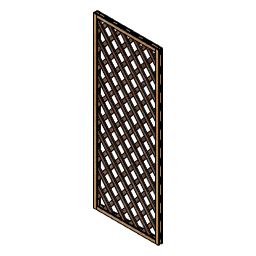
Latice Hanger (Autodesk Fusion 360 archive; units mm, degrees)
design "Lattice Wall"
Autodesk Fusion 360 part; units mm, degrees
sketch "Sketch1" plane through (0, 0, 0) normal (0, 1, 0) x (1, 0, 0) in component "Front"
  line L0 (405, 1050) -> (-405, 1050)
  line L1 (-405, 1050) -> (-405, -1050)
  line L2 (-405, -1050) -> (405, -1050)
  line L3 (405, -1050) -> (405, 1050)
  line L4 (405, 1050) -> (-405, -1050) construction
  line L5 (-405, 1050) -> (405, -1050) construction
  line L6 (-366, -1050) -> (-366, 1050)
  line L7 (0, -1645) -> (0, 1420) construction
  line L8 (366, -1050) -> (366, 1050)
  line L9 (366, -1011) -> (-366, -1011)
  line L10 (-366, 1011) -> (366, 1011)
  dimension "d2" = 810
  dimension "d3" = 2100
  dimension "d4" = 39
  dimension "d9" = 39
  dimension "d10" = 39
  constraint horizontal L0
  constraint perpendicular L0 L1
  constraint parallel L0 L2
  constraint parallel L1 L3
  constraint coincident L4 origin
  constraint coincident L5 origin
  constraint coincident L2 L6.start
  constraint coincident L0 L6.end
  constraint perpendicular L0 L6
  constraint perpendicular L2 L7
  constraint symmetric L6.start L7 L8.start
  constraint symmetric L6.end L7 L8.end
  constraint coincident L8 L9.start
  constraint coincident L6 L9.end
  constraint perpendicular L6 L9
  constraint coincident L6 L10.start
  constraint coincident L8 L10.end
  constraint perpendicular L8 L10
  measures "d2" distance of L1.end L2.end
  measures "d3" distance of L0.end L1.end
  measures "d4" distance of L1 L6
  measures "d9" distance of L2 L9
  measures "d10" distance of L0 L10
extrude "Extrude1" add sketch "Sketch1" along normal blind 12 contours L0 L2 L3 L8 | L0 L1 L2 L6 makes body 1 at (-392, 0, -350) makes body 2 at (379, 0, 350) in component "Front"
extrude "Extrude2" add sketch "Sketch1" along normal blind 12 separate body contours L0 L6 L8 L10 | L2 L6 L8 L9 makes body 3 at (-122, 0, -1024) makes body 4 at (-122, 0, 1037) in component "Front"
sketch "Sketch1 (2)" plane through (0, 0, 0) normal (0, 1, 0) x (1, 0, 0) in component "Middle Front"
  line L0 (-366, -1050) -> (-366, 1050) construction
  line L1 (366, -1011) -> (-366, -1011) construction
  line L2 (366, -1050) -> (366, 1050) construction
  line L3 (-366, 1011) -> (366, 1011) construction
  line L4 (-397.4531, -1050) -> (405, -55.0052)
  line L5 (405, 7.1195) -> (-405, -997.2331)
  line L6 (405, -190.405) -> (-288.2545, -1050)
  line L7 (-238.1517, -1050) -> (405, -252.5296)
  line L8 (80.4512, -1050) -> (405, -647.5785)
  line L9 (405, -585.4539) -> (30.3483, -1050)
  line L10 (-78.8502, -1050) -> (405, -450.054)
  line L11 (405, -387.9294) -> (-128.9531, -1050)
  line L12 (405, -1050) -> (405, 1050)
  line L13 (-405, -1050) -> (405, -1050)
  line L14 (-405, 1050) -> (-405, -1050)
  line L15 (405, 1050) -> (-405, 1050)
  line L16 (239.7526, -1050) -> (405, -845.1029)
  line L17 (405, -782.9783) -> (189.6497, -1050)
  line L18 (405, 204.6439) -> (-405, -799.7087)
  line L19 (-405, -861.8333) -> (405, 142.5193)
  line L20 (405, 402.1683) -> (-405, -602.1842)
  line L21 (-405, -664.3088) -> (405, 340.0437)
  line L22 (405, 599.6928) -> (-405, -404.6598)
  line L23 (-405, -466.7844) -> (405, 537.5682)
  line L24 (405, 797.2172) -> (-405, -207.1353)
  line L25 (-405, -269.26) -> (405, 735.0926)
  line L26 (405, 994.7417) -> (-405, -9.6109)
  line L27 (-405, -71.7355) -> (405, 932.617)
  line L28 (290.2639, 1050) -> (-405, 187.9135)
  line L29 (-405, 125.7889) -> (340.3667, 1050)
  line L30 (130.9624, 1050) -> (-405, 385.438)
  line L31 (-405, 323.3134) -> (181.0653, 1050)
  line L32 (-28.339, 1050) -> (-405, 582.9624)
  line L33 (-405, 520.8378) -> (21.7639, 1050)
  line L34 (-187.6404, 1050) -> (-405, 780.4869)
  line L35 (-405, 718.3622) -> (-137.5376, 1050)
  dimension "d15" = 39
  dimension "d16" = 39
  dimension "d17" = 85
  dimension "d18" = 39
  dimension "d19" = 39
  dimension "d20" = 85
  dimension "d21" = 85
  dimension "d22" = 39
  dimension "d23" = 85
  dimension "d24" = 39
  dimension "d25" = 39
  dimension "d26" = 39
  dimension "d27" = 39
  dimension "d28" = 39
  dimension "d29" = 39
  dimension "d30" = 39
  dimension "d31" = 39
  dimension "d32" = 39
  dimension "d33" = 85
  dimension "d34" = 85
  dimension "d35" = 85
  dimension "d36" = 85
  dimension "d37" = 85
  dimension "d38" = 85
  dimension "d39" = 85
  dimension "d40" = 85
  dimension "d41" = 85
  constraint parallel L4 L5
  constraint parallel L6 L7
  constraint parallel L10 L11
  constraint parallel L8 L9
  constraint coincident L12 L8.end
  constraint coincident L12 L9.start
  constraint coincident L12 L10.end
  constraint coincident L12 L11.start
  constraint coincident L12 L7.end
  constraint coincident L12 L6.start
  constraint coincident L12 L4.end
  constraint coincident L12 L5.start
  constraint coincident L14 L5.end
  constraint coincident L13 L4.start
  constraint coincident L13 L6.end
  constraint coincident L13 L7.start
  constraint coincident L13 L10.start
  constraint coincident L13 L11.end
  constraint coincident L13 L9.end
  constraint coincident L13 L8.start
  constraint parallel L16 L17
  constraint coincident L12 L17.start
  constraint coincident L12 L16.end
  constraint coincident L13 L16.start
  constraint coincident L13 L17.end
  constraint parallel L18 L19
  constraint parallel L20 L21
  constraint parallel L22 L23
  constraint parallel L24 L25
  constraint parallel L26 L27
  constraint parallel L28 L29
  constraint parallel L30 L31
  constraint parallel L32 L33
  constraint parallel L34 L35
  constraint coincident L15 L35.end
  constraint coincident L15 L34.start
  constraint coincident L15 L32.start
  constraint coincident L15 L33.end
  constraint coincident L15 L30.start
  constraint coincident L15 L31.end
  constraint coincident L15 L28.start
  constraint coincident L15 L29.end
  constraint coincident L12 L24.start
  constraint coincident L12 L25.end
  constraint coincident L14 L34.end
  constraint coincident L14 L35.start
  constraint coincident L14 L32.end
  constraint coincident L14 L33.start
  constraint coincident L14 L30.end
  constraint coincident L14 L31.start
  constraint coincident L14 L28.end
  constraint coincident L14 L29.start
  constraint coincident L14 L26.end
  constraint coincident L14 L22.end
  constraint coincident L14 L23.start
  constraint coincident L14 L20.end
  constraint coincident L14 L21.start
  constraint coincident L14 L18.end
  constraint coincident L14 L19.start
  constraint coincident L14 L25.start
  constraint coincident L14 L24.end
  constraint coincident L14 L27.start
  constraint coincident L12 L26.start
  constraint coincident L12 L27.end
  constraint coincident L12 L22.start
  constraint coincident L12 L23.end
  constraint coincident L12 L20.start
  constraint coincident L12 L21.end
  constraint coincident L12 L18.start
  constraint coincident L12 L19.end
  measures "d15" distance of L4 L5
  measures "d16" distance of L6 L7
  measures "d17" distance of L4 L6
  measures "d18" distance of L10 L11
  measures "d19" distance of L8 L9
  measures "d20" distance of L9 L10
  measures "d21" distance of L7 L11
  measures "d22" distance of L16 L17
  measures "d23" distance of L8 L17
  measures "d24" distance of L18 L19
  measures "d25" distance of L20 L21
  measures "d26" distance of L22 L23
  measures "d27" distance of L24 L25
  measures "d28" distance of L26 L27
  measures "d29" distance of L28 L29
  measures "d30" distance of L30 L31
  measures "d31" distance of L32 L33
  measures "d32" distance of L34 L35
  measures "d33" distance of L5 L19
  measures "d34" distance of L18 L21
  measures "d35" distance of L20 L23
  measures "d36" distance of L22 L25
  measures "d37" distance of L24 L27
  measures "d38" distance of L26 L29
  measures "d39" distance of L28 L31
  measures "d40" distance of L30 L33
  measures "d41" distance of L32 L35
extrude "Extrude1'" add sketch "Sketch1 (2)" along normal blind 13 separate body contours L4 L5 L12 L13 L14 | L6 L7 L12 L13 | L12 L14 L18 L19 | L10 L11 L12 L13 | L12 L14 L20 L21 | L8 L9 L12 L13 | L12 L14 L22 L23 | L12 L13 L16 L17 | L12 L14 L24 L25 | L12 L14 L26 L27 | L14 L15 L28 L29 | L14 L15 L30 L31 | L14 L15 L32 L33 | L14 L15 L34 L35 makes body 5 at (-209.6449, 0, -586.2504) makes body 6 at (135, 0, -244.2004) makes body 7 at (173.9152, 0, 497.6449) makes body 8 at (333.2166, 0, 892.6937) makes body 9 at (135, 0, 348.3729) makes body 10 at (135, 0, -441.7248) makes body 11 at (-262.7454, 0, -717.9334) makes body 12 at (-156.5444, 0, -454.5675) makes body 13 at (-135, 0, 308.8164) makes body 14 at (227.0156, 0, 629.3278) makes body 15 at (280.1161, 0, 761.0108) makes body 16 at (135, 0, 150.8485) makes body 17 at (135, 0, -639.2493) makes body 18 at (-315.8459, 0, -849.6164) in component "Middle Front"
sketch "Sketch1 (3)" plane through (0, 0, 0) normal (0, 1, 0) x (1, 0, 0) in component "Middle Back"
  line L0 (-366, -1050) -> (-366, 1050) construction
  line L1 (366, -1011) -> (-366, -1011) construction
  line L2 (366, -1050) -> (366, 1050) construction
  line L3 (-366, 1011) -> (366, 1011) construction
  line L4 (-397.4531, -1050) -> (405, -55.0052)
  line L5 (405, 7.1195) -> (-405, -997.2331)
  line L6 (405, -190.405) -> (-288.2545, -1050)
  line L7 (-238.1517, -1050) -> (405, -252.5296)
  line L8 (80.4512, -1050) -> (405, -647.5785)
  line L9 (405, -585.4539) -> (30.3483, -1050)
  line L10 (-78.8502, -1050) -> (405, -450.054)
  line L11 (405, -387.9294) -> (-128.9531, -1050)
  line L12 (405, -1050) -> (405, 1050)
  line L13 (-405, -1050) -> (405, -1050)
  line L14 (-405, 1050) -> (-405, -1050)
  line L15 (405, 1050) -> (-405, 1050)
  line L16 (239.7526, -1050) -> (405, -845.1029)
  line L17 (405, -782.9783) -> (189.6497, -1050)
  line L18 (405, 204.6439) -> (-405, -799.7087)
  line L19 (-405, -861.8333) -> (405, 142.5193)
  line L20 (405, 402.1683) -> (-405, -602.1842)
  line L21 (-405, -664.3088) -> (405, 340.0437)
  line L22 (405, 599.6928) -> (-405, -404.6598)
  line L23 (-405, -466.7844) -> (405, 537.5682)
  line L24 (405, 797.2172) -> (-405, -207.1353)
  line L25 (-405, -269.26) -> (405, 735.0926)
  line L26 (405, 994.7417) -> (-405, -9.6109)
  line L27 (-405, -71.7355) -> (405, 932.617)
  line L28 (290.2639, 1050) -> (-405, 187.9135)
  line L29 (-405, 125.7889) -> (340.3667, 1050)
  line L30 (130.9624, 1050) -> (-405, 385.438)
  line L31 (-405, 323.3134) -> (181.0653, 1050)
  line L32 (-28.339, 1050) -> (-405, 582.9624)
  line L33 (-405, 520.8378) -> (21.7639, 1050)
  line L34 (-187.6404, 1050) -> (-405, 780.4869)
  line L35 (-405, 718.3622) -> (-137.5376, 1050)
  dimension "d15_1" = 39
  dimension "d16_1" = 39
  dimension "d17_1" = 85
  dimension "d18_1" = 39
  dimension "d19_1" = 39
  dimension "d20_1" = 85
  dimension "d21_1" = 85
  dimension "d22_1" = 39
  dimension "d23_1" = 85
  dimension "d24_1" = 39
  dimension "d25_1" = 39
  dimension "d26_1" = 39
  dimension "d27_1" = 39
  dimension "d28_1" = 39
  dimension "d29_1" = 39
  dimension "d30_1" = 39
  dimension "d31_1" = 39
  dimension "d32_1" = 39
  dimension "d33_1" = 85
  dimension "d34_1" = 85
  dimension "d35_1" = 85
  dimension "d36_1" = 85
  dimension "d37_1" = 85
  dimension "d38_1" = 85
  dimension "d39_1" = 85
  dimension "d40_1" = 85
  dimension "d41_1" = 85
  constraint parallel L4 L5
  constraint parallel L6 L7
  constraint parallel L10 L11
  constraint parallel L8 L9
  constraint coincident L12 L8.end
  constraint coincident L12 L9.start
  constraint coincident L12 L10.end
  constraint coincident L12 L11.start
  constraint coincident L12 L7.end
  constraint coincident L12 L6.start
  constraint coincident L12 L4.end
  constraint coincident L12 L5.start
  constraint coincident L14 L5.end
  constraint coincident L13 L4.start
  constraint coincident L13 L6.end
  constraint coincident L13 L7.start
  constraint coincident L13 L10.start
  constraint coincident L13 L11.end
  constraint coincident L13 L9.end
  constraint coincident L13 L8.start
  constraint parallel L16 L17
  constraint coincident L12 L17.start
  constraint coincident L12 L16.end
  constraint coincident L13 L16.start
  constraint coincident L13 L17.end
  constraint parallel L18 L19
  constraint parallel L20 L21
  constraint parallel L22 L23
  constraint parallel L24 L25
  constraint parallel L26 L27
  constraint parallel L28 L29
  constraint parallel L30 L31
  constraint parallel L32 L33
  constraint parallel L34 L35
  constraint coincident L15 L35.end
  constraint coincident L15 L34.start
  constraint coincident L15 L32.start
  constraint coincident L15 L33.end
  constraint coincident L15 L30.start
  constraint coincident L15 L31.end
  constraint coincident L15 L28.start
  constraint coincident L15 L29.end
  constraint coincident L12 L24.start
  constraint coincident L12 L25.end
  constraint coincident L14 L34.end
  constraint coincident L14 L35.start
  constraint coincident L14 L32.end
  constraint coincident L14 L33.start
  constraint coincident L14 L30.end
  constraint coincident L14 L31.start
  constraint coincident L14 L28.end
  constraint coincident L14 L29.start
  constraint coincident L14 L26.end
  constraint coincident L14 L22.end
  constraint coincident L14 L23.start
  constraint coincident L14 L20.end
  constraint coincident L14 L21.start
  constraint coincident L14 L18.end
  constraint coincident L14 L19.start
  constraint coincident L14 L25.start
  constraint coincident L14 L24.end
  constraint coincident L14 L27.start
  constraint coincident L12 L26.start
  constraint coincident L12 L27.end
  constraint coincident L12 L22.start
  constraint coincident L12 L23.end
  constraint coincident L12 L20.start
  constraint coincident L12 L21.end
  constraint coincident L12 L18.start
  constraint coincident L12 L19.end
  measures "d15_1" distance of L4 L5
  measures "d16_1" distance of L6 L7
  measures "d17_1" distance of L4 L6
  measures "d18_1" distance of L10 L11
  measures "d19_1" distance of L8 L9
  measures "d20_1" distance of L9 L10
  measures "d21_1" distance of L7 L11
  measures "d22_1" distance of L16 L17
  measures "d23_1" distance of L8 L17
  measures "d24_1" distance of L18 L19
  measures "d25_1" distance of L20 L21
  measures "d26_1" distance of L22 L23
  measures "d27_1" distance of L24 L25
  measures "d28_1" distance of L26 L27
  measures "d29_1" distance of L28 L29
  measures "d30_1" distance of L30 L31
  measures "d31_1" distance of L32 L33
  measures "d32_1" distance of L34 L35
  measures "d33_1" distance of L5 L19
  measures "d34_1" distance of L18 L21
  measures "d35_1" distance of L20 L23
  measures "d36_1" distance of L22 L25
  measures "d37_1" distance of L24 L27
  measures "d38_1" distance of L26 L29
  measures "d39_1" distance of L28 L31
  measures "d40_1" distance of L30 L33
  measures "d41_1" distance of L32 L35
extrude "Extrude1''" add sketch "Sketch1 (3)" along normal blind 13 separate body contours L4 L5 L12 L13 L14 | L6 L7 L12 L13 | L12 L14 L18 L19 | L10 L11 L12 L13 | L12 L14 L20 L21 | L8 L9 L12 L13 | L12 L14 L22 L23 | L12 L13 L16 L17 | L12 L14 L24 L25 | L12 L14 L26 L27 | L14 L15 L28 L29 | L14 L15 L30 L31 | L14 L15 L32 L33 | L14 L15 L34 L35 makes body 19 at (-209.6449, 0, -586.2504) makes body 20 at (135, 0, -244.2004) makes body 21 at (173.9152, 0, 497.6449) makes body 22 at (333.2166, 0, 892.6937) makes body 23 at (135, 0, 348.3729) makes body 24 at (135, 0, -441.7248) makes body 25 at (-262.7454, 0, -717.9334) makes body 26 at (-156.5444, 0, -454.5675) makes body 27 at (-135, 0, 308.8164) makes body 28 at (227.0156, 0, 629.3278) makes body 29 at (280.1161, 0, 761.0108) makes body 30 at (135, 0, 150.8485) makes body 31 at (135, 0, -639.2493) makes body 32 at (-315.8459, 0, -849.6164) in component "Middle Back"
component "Frame" placed x (1, 0, 0) y (0, 1, 0) z (0, 0, 1) at (0, 0, 0)
component "Front" placed x (1, 0, 0) y (0, 1, 0) z (0, 0, 1) at (0, -10, 0) in component "Frame"
component "Middle Front" placed x (1, 0, 0) y (0, 1, 0) z (0, 0, 1) at (0, 0, 0) in component "Frame"
component "Middle Back" placed x (-1, 0, 0) y (0, -1, 0) z (0, 0, 1) at (0.6358, 26, 0) in component "Frame"
component "Front" placed x (1, 0, 0) y (0, 1, 0) z (0, 0, 1) at (0, 25, 0) in component "Frame"
equation "d9 = d4"
equation "d10 = d9"
